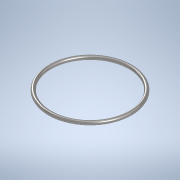
# Autodesk Inventor part: Пружина дросселя
Saved by Autodesk Inventor 2021 (Build 250183000, 183)
## iProperties
Created: 2020-11-05
Part Number: Пружина дросселя
Material: Сталь, углеродистая
Document SubType Name: Modeling
Designer: Тимоха
Density: 7.85 g/cm^3
Appearance: С умеренной полировкой
Mass: 26.6519 g
Surface Area: 33.9514 cm^2
Volume: 3.39514 cm^3
Author: Тимоха
Autodesk Inventor part; units mm, degrees
ref_plane "YZ Plane" through (0, 0, 0) normal (1, 0, 0) x (0, 1, 0)
ref_plane "XZ Plane" through (0, 0, 0) normal (0, 1, 0) x (-1, 0, 0)
ref_plane "XY Plane" through (0, 0, 0) normal (0, 0, 1) x (1, 0, 0)
sketch "Эскиз1" plane through (0, 0, 0) normal (0, 0, 1) x (1, 0, 0)
  line L0 (0, 0) -> (43, 0)
  circle A0 centre (43, 0) radius 2
  line L1 (0, -2.8) -> (0, 2.8) projected
  dimension "d0" = 43
  dimension "d1" = 4
  constraints: 2 end point, 1 centre point, 1 coincident, 1 horizontal
  measures "d0" distance of L0.start L0.end
  measures "d1" diameter of A0
revolve "Вращение1" add sketch "Эскиз1" angle 360 about axis through (0, -10, 0) along (0, 1, 0)
